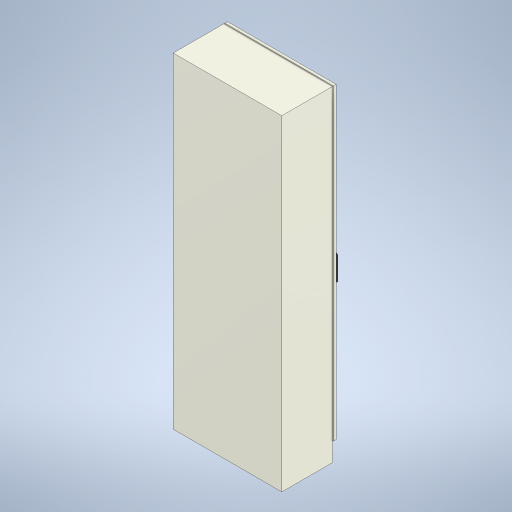
# Autodesk Inventor part: Schaltschrank1
Saved by Autodesk Inventor 2023 (Build 270158000, 158)
## iProperties
Created: 2025-06-27
Part Number: Schaltschrank1
Material: Generisch
Document SubType Name: Modeling
Designer: aurich
Density: 1 g/cm^3
Appearance: Vorgabe
Author: aurich
Autodesk Inventor part; units mm, degrees
ref_plane "YZ Plane" through (0, 0, 0) normal (1, 0, 0) x (0, 1, 0)
ref_plane "XZ Plane" through (0, 0, 0) normal (0, 1, 0) x (-1, 0, 0)
ref_plane "XY Plane" through (0, 0, 0) normal (0, 0, 1) x (1, 0, 0)
sketch "Skizze1" plane through (0, 0, 0) normal (0, 1, 0) x (-1, 0, 0)
  line L0 (0, 0) -> (600, 0)
  line L1 (600, 0) -> (600, -280)
  line L2 (600, -280) -> (0, -280)
  line L3 (0, -280) -> (0, 0)
  dimension "d0" = 600
  dimension "d1" = 280
  constraints: 8 end point, 2 parallel, 1 horizontal, 1 perpendicular
  measures "d0" distance of L1.end L2.end
  measures "d1" distance of L0.end L1.end
extrude "Extrusion1" add sketch "Skizze1" along normal blind 1800
sketch "Skizze2" plane through (0, 0, -280) normal (0, 0, -1) x (-1, 0, 0)
  line L0 (10, 1790) -> (590, 1790)
  line L1 (590, 1790) -> (590, 110)
  line L2 (590, 110) -> (10, 110)
  line L3 (10, 110) -> (10, 1790)
  line L4 (0, 0) -> (0, 1800) projected
  line L5 (600, 0) -> (600, 1800) projected
  line L6 (0, 1800) -> (600, 1800) projected
  line L7 (0, 0) -> (600, 0) projected
  dimension "d4" = 10
  dimension "d5" = 10
  dimension "d6" = 10
  dimension "d7" = 110
  constraints: 8 end point, 2 parallel, 1 horizontal, 1 perpendicular
  measures "d4" distance between parallel lines of L4 L3
  measures "d5" distance between parallel lines of L1 L5
  measures "d6" distance between parallel lines of L6 L0
  measures "d7" distance between parallel lines of L7 L2
extrude "Extrusion2" add sketch "Skizze2" along normal blind 5 contours L0 L1 L2 L3
sketch "Skizze3" plane through (0, 0, -285) normal (0, 0, -1) x (-1, 0, 0)
  line L0 (0, 0) -> (0, 1800) projected
  line L1 (600, 0) -> (600, 1800) projected
  line L2 (0, 1800) -> (600, 1800)
  line L3 (600, 1800) -> (600, 100)
  line L4 (600, 100) -> (0, 100)
  line L5 (0, 100) -> (0, 1800)
  line L6 (10, 110) -> (590, 110) projected
  point P0 (0, 100)
  dimension "d10" = 10
  constraints: 8 end point, 2 parallel, 1 horizontal, 1 perpendicular, 1 point on line
  measures "d10" distance between parallel lines of L4 L6
extrude "Extrusion3" add sketch "Skizze3" along normal blind 15
sketch "Skizze4" plane through (0, 0, -300) normal (0, 0, -1) x (-1, 0, 0)
  line L0 (15, 980) -> (25, 980)
  line L1 (35, 970) -> (35, 850)
  line L2 (25, 840) -> (15, 840)
  line L3 (5, 850) -> (5, 970)
  line L4 (0, 0) -> (600, 0) projected
  line L5 (0, 1800) -> (0, 100) projected
  arc A0 (5, 850) -> (15, 840) centre (15, 850) ccw
  arc A1 (25, 840) -> (35, 850) centre (25, 850) ccw
  arc A2 (35, 970) -> (25, 980) centre (25, 970) ccw
  arc A3 (15, 980) -> (5, 970) centre (15, 970) ccw
  dimension "d13" = 840
  dimension "d14" = 140
  dimension "d15" = 30
  dimension "d16" = 5
  dimension "d17" = 10
  constraints: 8 end point, 8 point on circle, 8 tangent, 4 centre point, 3 equal radius, 2 parallel, 1 horizontal, 1 perpendicular
  measures "d13" distance between parallel lines of L4 L2
  measures "d14" distance between parallel lines of L0 L2
  measures "d15" distance between parallel lines of L1 L3
  measures "d16" distance between parallel lines of L3 L5
  measures "d17" radius of A0
extrude "Extrusion4" add sketch "Skizze4" along normal blind 15
equation "\"d5\" = d4"
equation "\"d6\" = d5"
